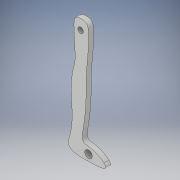
# Autodesk Inventor part: pierna
Saved by Autodesk Inventor 2019 (Build 230136000, 136)
## iProperties
Created: 2019-11-15
Part Number: pierna
Material: Generic
Document SubType Name: Modeling
Designer: Domenico
Density: 1 g/cm^3
Appearance: Default
Author: Domenico
Autodesk Inventor part; units mm, degrees
ref_plane "YZ Plane" through (0, 0, 0) normal (1, 0, 0) x (0, 1, 0)
ref_plane "XZ Plane" through (0, 0, 0) normal (0, 1, 0) x (-1, 0, 0)
ref_plane "XY Plane" through (0, 0, 0) normal (0, 0, 1) x (1, 0, 0)
sketch "Sketch1" plane through (0, 0, 0) normal (0, 0, 1) x (1, 0, 0)
  circle A0 centre (0, 0) radius 6.7
  line L0 (0, 0) -> (-28.26, 0) construction
  line L1 (-28.26, 0) -> (-28.26, 186) construction
  line L2 (-28.26, 186) -> (-14.13, 186) construction
  circle A1 centre (-14.13, 186) radius 5
  line L3 (27.575, 0) -> (20.5132, 6.7) construction
  line L4 (20.5132, 6.7) -> (6.7, 11.0766) construction
  line L5 (6.7, 11.0766) -> (-3.8106, 13.0382) construction
  line L6 (-3.8106, 13.0382) -> (-9.13, 13.0382) construction
  line L7 (-9.13, 13.0382) -> (-11.2647, 18.5306) construction
  line L8 (-11.2647, 18.5306) -> (-11.2647, 23.6308) construction
  line L9 (-11.2647, 23.6308) -> (-9.13, 38.5389) construction
  line L10 (-9.13, 38.5389) -> (-6.7, 52.6624) construction
  line L11 (-6.7, 52.6624) -> (-4.2029, 79.3402) construction
  line L12 (-4.2029, 79.3402) -> (-4.2029, 103.664) construction
  line L13 (-4.2029, 103.664) -> (-4.2029, 129.5571) construction
  line L14 (-4.2029, 129.5571) -> (0, 158.981) construction
  line L15 (0, 158.981) -> (0, 186) construction
  line L16 (0, 186) -> (0, 200.1746) construction
  line L17 (0, 200.1746) -> (-6.7, 204.8824) construction
  line L18 (-6.7, 204.8824) -> (-19.13, 204.8824) construction
  line L19 (-19.13, 204.8824) -> (-26.1728, 199.39) construction
  line L20 (-26.1728, 199.39) -> (-26.1728, 191) construction
  line L21 (-26.1728, 191) -> (-26.1728, 177.0277) construction
  line L22 (-26.1728, 177.0277) -> (-23.8189, 145.2499) construction
  line L23 (-23.8189, 145.2499) -> (-23.8189, 128.7724) construction
  line L24 (-23.8189, 128.7724) -> (-28.26, 120.8239) construction
  line L25 (-28.26, 120.8239) -> (-31.273, 97.4396) construction
  line L26 (-31.273, 97.4396) -> (-31.273, 71.5421) construction
  line L27 (-31.273, 71.5421) -> (-28.26, 47.5623) construction
  line L28 (-28.26, 47.5623) -> (-30.8806, 21.2769) construction
  line L29 (-30.8806, 21.2769) -> (-34.8038, 6.7) construction
  line L30 (-34.8038, 6.7) -> (-38.727, 0) construction
  line L31 (-38.727, 0) -> (-31.273, -11.2856) construction
  line L32 (-31.273, -11.2856) -> (-9.13, -11.2856) construction
  line L33 (-9.13, -11.2856) -> (25.6134, -11.2856) construction
  line L34 (25.6134, -11.2856) -> (35.029, -6.7) construction
  line L35 (35.029, -6.7) -> (27.575, 0) construction
  spline S0 degree 4 poles (27.575, 0) (20.5132, 6.7) (6.7, 11.0766) (-3.8106, 13.0382) (-9.13, 13.0382) (-11.2647, 18.5306) (-11.2647, 23.6308) (-9.13, 38.5389) (-6.7, 52.6624) (-4.2029, 79.3402) (-4.2029, 103.664) (-4.2029, 129.5571) (0, 158.981) (0, 186) (0, 200.1746) (-6.7, 204.8824) (-19.13, 204.8824) (-26.1728, 199.39) (-26.1728, 191) (-26.1728, 177.0277) (-23.8189, 145.2499) (-23.8189, 128.7724) (-28.26, 120.8239) (-31.273, 97.4396) (-31.273, 71.5421) (-28.26, 47.5623) (-30.8806, 21.2769) (-34.8038, 6.7) (-38.727, 0) (-31.273, -11.2856) (-9.13, -11.2856) (25.6134, -11.2856) (35.029, -6.7) (27.575, 0) knots 1 1 1 1 1 2 3 4 5 6 7 8 9 10 11 12 13 14 15 16 17 18 19 20 21 22 23 24 25 26 27 28 29 30 31 31 31 31 31
  dimension "d0" = 13.4
  dimension "d1" = 28.26
  dimension "d2" = 186
  dimension "d3" = 10
  constraints: 6 end point, 6 vertical, 4 horizontal, 3 parallel, 3 perpendicular, 2 centre point, 2 coincident, 2 point on line, 2 other
  measures "d0" diameter of A0
  measures "d1" distance of L0.start L0.end
  measures "d2" distance of L0.end L1.end
  measures "d3" diameter of A1
extrude "Extrusion1" add sketch "Sketch1" along normal blind 9
body "Solid1"
